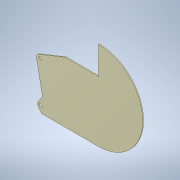
# Autodesk Inventor part: 回路BOX側面
Saved by Autodesk Inventor 2020.2 (Build 242310000, 310)
## iProperties
Created: 2020-03-29
Part Number: 回路BOX側面
Material: ポリプロピレン
Document SubType Name: Modeling
Designer: aoyama
Density: 0.899 g/cm^3
Appearance: 滑らか - 灰色
Mass: 3.58483 g
Surface Area: 108.894 cm^2
Volume: 3.98757 cm^3
Author: aoyama
Autodesk Inventor part; units mm, degrees
ref_plane "YZ Plane" through (0, 0, 0) normal (1, 0, 0) x (0, 1, 0)
ref_plane "XZ Plane" through (0, 0, 0) normal (0, 1, 0) x (-1, 0, 0)
ref_plane "XY Plane" through (0, 0, 0) normal (0, 0, 1) x (1, 0, 0)
sketch "スケッチ1" plane through (0, 0, 0) normal (0, 0, 1) x (1, 0, 0)
  line L0 (44.9825, 3) -> (44.9825, 0) construction
  line L1 (44.9825, 0) -> (93.5151, 0) construction
  line L2 (44.9825, 3) -> (93.5151, 3) construction
  circle A0 centre (152.1179, -73.6808) radius 5 construction
  circle A1 centre (90.7937, -5.925) radius 3 construction
  circle A2 centre (91.5613, -41.579) radius 3 construction
  line L3 (50.9825, 0) -> (47.9825, 0) construction
  line L4 (47.9825, 0.7) -> (50.9825, 0.7) construction
  circle A3 centre (110.1553, -43.629) radius 14 construction
  circle A4 centre (105.6122, -16) radius 14 construction
  arc A5 (39.4825, -0.75) -> (39.4825, -77.9308) centre (39.4825, -39.3404) ccw construction
  line L5 (-44.9825, -3) -> (-44.9825, 0)
  line L6 (-44.9825, 0) -> (-93.5151, 0)
  line L7 (-44.9825, -3) -> (-93.5151, -3)
  circle A6 centre (-152.1179, 73.6808) radius 5
  circle A7 centre (-90.7937, 5.925) radius 3
  circle A8 centre (-91.5613, 41.579) radius 3
  line L8 (-50.9825, 0) -> (-47.9825, 0)
  line L9 (-47.9825, -0.7) -> (-50.9825, -0.7)
  circle A9 centre (-110.1553, 43.629) radius 14
  circle A10 centre (-105.6122, 16) radius 14
  arc A11 (-39.4825, 0.75) -> (-39.4825, 77.9308) centre (-39.4825, 39.3404) ccw
  line L10 (-97.013, 53.9033) -> (-2.9368, 53.9033)
  circle A12 centre (-91.5613, 41.579) radius 1.5
  circle A13 centre (-90.7937, 5.925) radius 1.5
  line L11 (-97.013, 53.9033) -> (-89.1899, 13.6565)
  line L12 (-89.1899, 13.6565) -> (-98.7082, -0.429)
  line L13 (0, 0) -> (-132.2518, 0)
  line L14 (-98.4183, 0) -> (-39.4825, 0)
  arc A14 (-39.4825, 0) -> (-39.4825, 78.6808) centre (-39.4825, 39.3404) ccw
  line L15 (-39.4825, 78.6808) -> (-39.4825, 53.9033)
  line L16 (-94.9784, 43.4362) -> (-69.0084, 53.9033)
  line L17 (-92.9751, 3.8654) -> (-89.8036, 0)
  point P0 (49.4825, 0.7)
  point P1 (-49.4825, -0.7)
  point P2 (-39.4825, 0)
  point P3 (-39.4825, 78.6808)
  point P4 (-92.6828, 44.3615)
  point P5 (-94.5062, 41.0065)
  point P6 (-44.9825, 0)
  point P7 (-89.8036, 0)
  point P8 (-93.2794, 7.6047)
  dimension "d2" = 360
  dimension "d4" = 3
  dimension "d5" = 3
  dimension "d6" = 1.5
  dimension "d7" = 41
  dimension "d8" = 79
  dimension "d9" = 17
  dimension "d11" = 0.75
  dimension "d14" = 28
  dimension "d16" = 5
  constraints: 36 end point, 14 centre point, 8 point on line, 7 point on circle, 6 horizontal, 2 coincident, 2 tangent, 1 vertical, 84 other
  measures "d4" diameter of A12
  measures "d5" diameter of A13
  measures "d6" radial gap between concentric circles of A8 A12
  measures "d7" distance of L10.start L11.end
  measures "d8" angle of L10 L11
  measures "d9" distance of L11.end L12.end
  measures "d11" radial gap between concentric circles of A11 A14
  measures "d14" distance of L16.start L16.end
  measures "d16" distance of L17.start L17.end
extrude "押し出し1" add sketch "スケッチ1" along normal blind 0.75 contours L6 L17 A7 L12 L11 A8 L16 L10 A14 L13 | L10 A11 L15 A14 | L10 L15 A11 | A7 | A8
